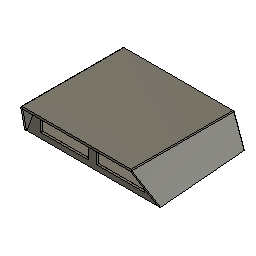
double auber gauge holder (Autodesk Fusion 360 design; units mm, degrees)
Autodesk Fusion 360 part; units mm, degrees
sketch "Sketch1" plane through (0, 0, 0) normal (0, 0, 1) x (1, 0, 0)
  line L0 (14.9145, 27.5) -> (59.9145, 27.5)
  line L1 (59.9145, 27.5) -> (59.9145, 5)
  line L2 (59.9145, 5) -> (14.9145, 5)
  line L3 (14.9145, 5) -> (14.9145, 27.5)
  line L4 (0, 0) -> (11.829, 32.5)
  line L5 (11.829, 32.5) -> (116, 32.5)
  line L6 (0, 0) -> (127.829, 0)
  line L7 (63.9145, 0) -> (63.9145, 46.8589) construction
  line L8 (67.9145, 5) -> (112.9145, 5)
  line L9 (112.9145, 5) -> (112.9145, 27.5)
  line L10 (67.9145, 27.5) -> (67.9145, 5)
  line L11 (112.9145, 27.5) -> (67.9145, 27.5)
  line L12 (127.829, 0) -> (116, 32.5)
  line L13 (0, 0) -> (0, 5)
  line L14 (0, 5) -> (14.9145, 5)
  point P0 (121.9145, 16.25)
  dimension "d1" = 45
  dimension "d2" = 22.5
  dimension "d6" = 5
  dimension "d7" = 8
  dimension "d8" = 70
  dimension "d9" = 5
  dimension "d10" = 9
  constraint horizontal L0
  constraint vertical L1
  constraint horizontal L2
  constraint vertical L3
  constraint coincident L4.start L6.start
  constraint horizontal L5
  constraint horizontal L6
  constraint coincident L6 L7.start
  constraint perpendicular L6 L7
  constraint symmetric L0.start L7 L9.end
  constraint symmetric L0.end L7 L10.start
  constraint symmetric L1.end L7 L8.start
  constraint symmetric L2.end L7 L8.end
  constraint symmetric L4.start L7 L6.end
  constraint symmetric L4.end L7 L5.end
  constraint coincident L5.end L12.end
  constraint midpoint L12 P0
  constraint perpendicular L6 L13
  measures "d1" distance of L0.start L0.end
  measures "d2" distance of L0.start L2.end
  measures "d6" vertical distance of L4.start L2.end
  measures "d7" distance of L1 L10
  measures "d8" angle of L6 L12
  measures "d9" distance of L5 L11
  measures "d10" distance of L9 P0
sketch "Sketch2" plane through (0, 0, 0) normal (1, 0, 0) x (0, 0, -1)
  line L0 (0, 5) -> (78, 5)
  line L1 (0, 0) -> (78, 5)
  line L2 (0, 27.5) -> (77.9984, 27)
  line L3 (0, 32.5) -> (80.5732, 32.5)
  line L4 (78, 5) -> (98.5779, 6.3191)
  line L5 (80.5732, 32.5) -> (98.5779, 6.3191)
  line L6 (0, 32.5) -> (2, 32.5)
  line L7 (2, 32.5) -> (2, 0.1282)
  line L8 (0, 0) -> (0, 32.5)
  line L9 (0, 32.5) -> (80.8342, 32.5)
  line L10 (80.8342, 32.5) -> (80.8342, 30.5)
  line L11 (80.8342, 30.5) -> (0, 30.5)
  line L12 (0, 30.5) -> (0, 32.5)
  line L13 (98.5779, 6.3191) -> (111.5874, -12.5984)
  line L14 (111.5874, -12.5984) -> (0, -12.5984)
  line L15 (0, -12.5984) -> (0, 0)
  line L16 (2, 2.25) -> (35.1, 2.25)
  line L17 (0, 4.25) -> (66.3, 4.25)
  line L18 (2, 2.25) -> (0, 2.25)
  point P0 (0, 5)
  point P1 (0, 27.5)
  point P2 (0, 32.5)
  dimension "d11" = 78
  dimension "d12" = 78
  dimension "d15" = 2
  dimension "d16" = 2
  dimension "d25" = 2.75
  dimension "d26" = 2
  constraint horizontal L0
  constraint coincident P0 L0.start
  constraint coincident L1.start L8.start
  constraint coincident P1 L2.start
  constraint coincident P2 L3.start
  constraint horizontal L3
  constraint parallel L1 L4
  constraint horizontal L6
  constraint vertical L7
  constraint vertical L8
  constraint horizontal L9
  constraint vertical L10
  constraint horizontal L11
  constraint vertical L12
  constraint parallel L5 L13
  constraint horizontal L14
  constraint parallel L7 L15
  constraint coincident L7 L16.start
  constraint perpendicular L7 L16
  constraint coincident L8 L17.start
  constraint perpendicular L8 L17
  constraint coincident L1 L16.end
  constraint coincident L1 L17.end
  constraint coincident L8 L18.end
  constraint perpendicular L8 L18
  constraint coincident L1 L7.end
  measures "d11" distance of P0 L0.end
  measures "d12" distance of P1 L2.end
  measures "d15" distance of P2 L6.end
  measures "d16" distance of P2 L11.end
  measures "d25" distance of L0 L16
  measures "d26" distance of L16 L17
extrude "Extrude1" add sketch "Sketch1" against normal blind 2 contours L4 L5 L6 L12
extrude "Extrude2" cut sketch "Sketch2" along normal blind 170 contours L1 L4 L13 L14 L15
extrude "Extrude3" add 1 faces at (117.8705, 10.8761, -2) along direction (0, 0, -1) blind 80 thin wall 2 inside
extrude "Extrude4" cut 2 faces at (44.9145, 3.6667, -82) (97.9145, 3.6667, -82) along direction (0, 0, -1) up to surface end surface through (0, 0, -2) normal (0, 0, -1) offset 0
extrude "Extrude5" cut sketch "Sketch2" along normal blind 180 contours L1 L4 L13 L14 L15
extrude "Extrude6" add sketch "Sketch2" along normal blind 125 contours L7 L8 L17 L18 | L1 L7 L16 L17 | L1 L7 L8 L18 | L1 L7 L16
extrude "Extrude7" cut sketch "Sketch1" against normal blind 280 contours L4 L13 L14
fillet "Fillet1" radius 1 5 edges at (116, 32.5, -41) (11.829, 32.5, -41) (6.8711, 18.8782, -82) (63.9145, 32.5, -82) (120.9579, 18.8782, -82)
sketch "Sketch3" plane through (0, 4.25, 0) normal (0, 1, 0) x (-1, 0, 0)
  line L0 (-124.1538, -2) -> (-124.1538, -66.3)
  line L1 (-124.1538, -66.3) -> (-3.6752, -66.3)
  line L2 (-3.6752, -66.3) -> (-3.6752, -2)
  line L3 (-3.6752, -2) -> (-124.1538, -2)
  line L4 (-124.1538, -66.3) -> (-124.1538, -2)
  line L5 (-3.6752, -2) -> (-3.6752, -66.3)
  line L6 (-124.1538, -66.3) -> (-3.6752, -66.3)
  line L7 (-3.6752, -66.3) -> (-3.6752, -34.15)
  line L8 (-3.6752, -34.15) -> (-124.1538, -34.15)
  line L9 (-124.1538, -34.15) -> (-124.1538, -66.3)
  constraint horizontal L6
  constraint vertical L7
  constraint horizontal L8
  constraint vertical L9
  constraint midpoint L5 L7.end
  constraint coincident L0.end L1.start
extrude "Extrude8" cut sketch "Sketch3" against normal blind 20 contours L0 L1 L2 L4 L5 L6 L7 L8 L9
sketch "Sketch4" plane through (0, 0, 0) normal (0, 0, 1) x (1, 0, 0)
  arc A0 (12.5292, 32.5) -> (11.5895, 31.842) centre (12.5292, 31.5) ccw
  line L0 (11.5895, 31.842) -> (0, 0)
  line L1 (0, 0) -> (127.829, 0)
  line L2 (127.829, 0) -> (116.2395, 31.842)
  arc A1 (116.2395, 31.842) -> (115.2998, 32.5) centre (115.2998, 31.5) ccw
  line L3 (115.2998, 32.5) -> (12.5292, 32.5)
  line L4 (67.9145, 27.5) -> (112.9145, 27.5)
  line L5 (112.9145, 27.5) -> (112.9145, 5)
  line L6 (112.9145, 5) -> (67.9145, 5)
  line L7 (67.9145, 5) -> (67.9145, 27.5)
  line L8 (59.9145, 5) -> (14.9145, 5)
  line L9 (14.9145, 5) -> (14.9145, 27.5)
  line L10 (14.9145, 27.5) -> (59.9145, 27.5)
  line L11 (59.9145, 27.5) -> (59.9145, 5)
  line L12 (124.9727, 2) -> (114.5996, 30.5)
  line L13 (114.5996, 30.5) -> (13.2294, 30.5)
  line L14 (13.2294, 30.5) -> (2.8563, 2)
  line L15 (2.8563, 2) -> (2.1284, 0)
  line L16 (13.2294, 30.5) -> (13.9574, 32.5)
  line L17 (114.5996, 30.5) -> (113.8716, 32.5)
  line L18 (124.9727, 2) -> (125.7007, 0)
  line L19 (114.5996, 30.5) -> (116.7279, 30.5)
  line L20 (13.2294, 30.5) -> (11.1011, 30.5)
  constraint coincident L1 L15.end
  constraint parallel L14 L15
  constraint coincident L3 L16.end
  constraint parallel L14 L16
  constraint coincident L3 L17.end
  constraint parallel L12 L17
  constraint coincident L1 L18.end
  constraint parallel L12 L18
  constraint coincident L2 L19.end
  constraint parallel L13 L19
  constraint coincident L0 L20.end
  constraint parallel L13 L20
extrude "Extrude9" add sketch "Sketch4" along normal blind 15 contours A0 L0 L3 L16 L20 | L3 L13 L16 L17 | L0 L1 L14 L15 L20 | L2 A1 L3 L17 L19 | L1 L2 L12 L18 L19
sketch "Sketch5" plane through (1.8794, -0.684, 0) normal (0.939693, -0.34202, 0) x (0, 0, -1)
  line L0 (0, 0.7279) -> (0, 33.1854)
  line L1 (0, 33.1854) -> (-15, 33.1854)
  line L2 (-15, 33.1854) -> (-15, 0.7279)
  line L3 (-15, 0.7279) -> (0, 0.7279)
  line L4 (0, 0) -> (-15, 33.1854)
  constraint coincident L4.start origin
  constraint coincident L1.end L2.start
extrude "Extrude10" cut sketch "Sketch5" against normal blind 30 contours L2 L3 L4
extrude "Extrude11" cut 1 faces at (0.8754, 0.456, 5.2194) along direction (-0.34202, -0.939693, 0) blind 12
sketch "Sketch6" plane through (110.9965, 40.3994, 0) normal (-0.939693, -0.34202, 0) x (0, 0, 1)
  line L0 (0, -10.5347) -> (0, -42.9922)
  line L1 (0, -42.9922) -> (15, -42.9922)
  line L2 (15, -42.9922) -> (15, -10.5347)
  line L3 (15, -10.5347) -> (0, -10.5347)
sketch "Sketch7" plane through (110.9965, 40.3994, 0) normal (-0.939693, -0.34202, 0) x (0, 0, 1)
  line L0 (0, -43) -> (15, -10.5347)
  line L1 (0, -10.5347) -> (0, -42.9922)
  line L2 (0, -42.9922) -> (15, -42.9922)
  line L3 (15, -42.9922) -> (15, -10.5347)
  line L4 (15, -10.5347) -> (0, -10.5347)
  constraint coincident L0.end L3.end
extrude "Extrude12" cut sketch "Sketch7" against normal blind 16 contours L0 L2 L3
extrude "Extrude13" cut 1 faces at (126.3271, 0.228, 5.0024) along direction (0.34202, -0.939693, 0) blind 7
